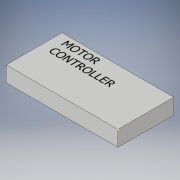
# Autodesk Inventor part: MotorController
Saved by Autodesk Inventor 2019 (Build 230136000, 136)
## iProperties
Created: 2019-06-19
Part Number: MotorController
Material: Generic
Document SubType Name: Modeling
Designer: abdel
Density: 1 g/cm^3
Appearance: Default
Author: abdel
Autodesk Inventor part; units mm, degrees
ref_plane "YZ Plane" through (0, 0, 0) normal (1, 0, 0) x (0, 1, 0)
ref_plane "XZ Plane" through (0, 0, 0) normal (0, 1, 0) x (-1, 0, 0)
ref_plane "XY Plane" through (0, 0, 0) normal (0, 0, 1) x (1, 0, 0)
sketch "Sketch1" plane through (0, 0, 0) normal (0, 1, 0) x (-1, 0, 0)
  line L0 (0, 0) -> (45.7911, 0)
  line L1 (45.7911, 0) -> (45.7911, -22.86)
  line L2 (45.7911, 0) -> (0, 0)
  line L3 (0, 0) -> (0, -22.86)
  line L4 (0, -22.86) -> (45.7911, -22.86)
  line L5 (45.7911, -22.86) -> (45.7911, 0)
  dimension "d0" = 45.7911
  dimension "d1" = 22.86
  constraints: 12 end point, 2 horizontal, 2 parallel, 2 perpendicular
  measures "d0" distance of L0.start L0.end
  measures "d1" distance of L0.end L1.end
extrude "Extrusion1" add sketch "Sketch1" along normal blind 6.35
sketch "Sketch2" plane through (0, 6.35, 0) normal (0, 1, 0) x (1, 0, 0)
  line L0 (-42.0648, 21.369) -> (-29.5251, 21.369) construction
  line L1 (-29.5251, 21.369) -> (-29.5251, 5.7143) construction
  line L2 (-29.5251, 5.7143) -> (-42.0648, 5.7143) construction
  line L3 (-42.0648, 5.7143) -> (-42.0648, 21.369) construction
  point P0 (0, 0)
  constraints: 2 other
body "Solid1"
